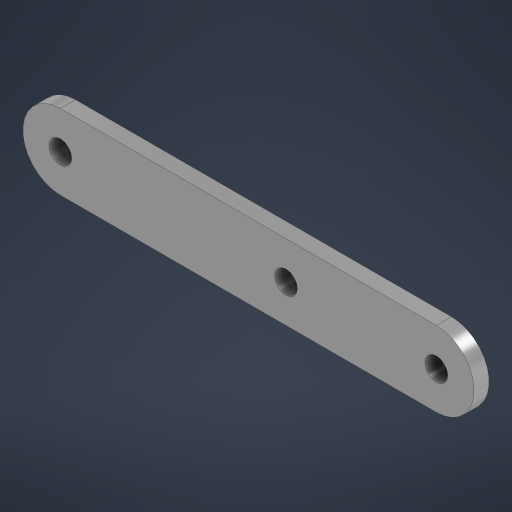
# Autodesk Inventor part: Side Support 2
Saved by Autodesk Inventor 2023 (Build 270158000, 158)
## iProperties
Created: 2023-04-12
Part Number: Side Support 2
Material: Generic
Document SubType Name: Modeling
Designer: vatdu
Density: 1 g/cm^3
Appearance: Default
Author: vatdu
Autodesk Inventor part; units mm, degrees
ref_plane "YZ Plane" through (0, 0, 0) normal (1, 0, 0) x (0, 1, 0)
ref_plane "XZ Plane" through (0, 0, 0) normal (0, 1, 0) x (-1, 0, 0)
ref_plane "XY Plane" through (0, 0, 0) normal (0, 0, 1) x (1, 0, 0)
sketch "Sketch1" plane through (0, 0, 0) normal (0, 0, 1) x (1, 0, 0)
  line L0 (0, 0) -> (60, 0)
  line L1 (60, 0) -> (60, 10)
  line L2 (60, 10) -> (0, 10)
  line L3 (0, 10) -> (0, 0)
  dimension "d0" = 60
  dimension "d1" = 10
  constraints: 8 end point, 2 parallel, 1 horizontal, 1 perpendicular
  measures "d0" distance of L2.end L1.end
  measures "d1" distance of L1.end L0.end
extrude "Extrusion1" add sketch "Sketch1" along normal blind 2
fillet "Fillet1" radius 5 4 edges at (0, 10, 1) (0, 0, 1) (60, 10, 1) (60, 0, 1)
sketch "Sketch2" plane through (0, 0, 2) normal (0, 0, 1) x (1, 0, 0)
  arc A0 (5, 10) -> (5, 0) centre (5, 5) ccw projected
  circle A1 centre (5, 5) radius 1.5
  arc A2 (55, 0) -> (55, 10) centre (55, 5) ccw projected
  circle A3 centre (55, 5) radius 1.5
  line L0 (55, 10) -> (5, 10) projected
  line L1 (30, 10) -> (30, 5)
  line L2 (30, 5) -> (35, 5)
  circle A4 centre (35, 5) radius 1.5
  point P0 (0, 0)
  dimension "d5" = 3
  dimension "d6" = 3
  dimension "d9" = 5
  dimension "d10" = 3
  constraints: 4 end point, 3 centre point, 3 coincident, 1 midpoint, 1 perpendicular, 1 vertical
  measures "d5" diameter of A1
  measures "d6" diameter of A3
  measures "d9" distance of L1.end L2.end
  measures "d10" diameter of A4
extrude "Extrusion2" cut sketch "Sketch2" against normal blind 2
body "Solid1"
